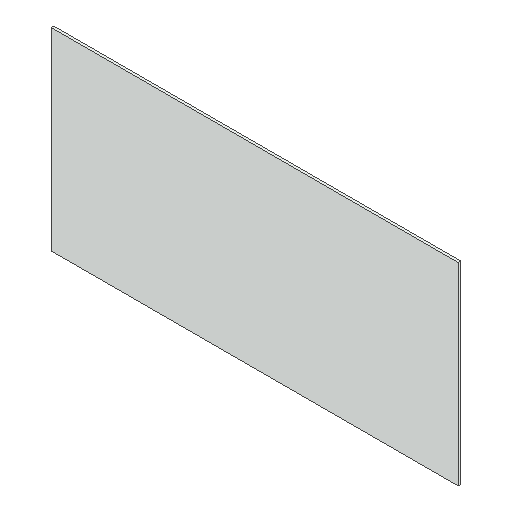
# Autodesk Inventor part: Chapa Frontal - Intake
Saved by Autodesk Inventor 2027.1 (Build 311270010, 270A)
## iProperties
Created: 2026-05-13
Part Number: Chapa Frontal - Intake
Material: Genérico
Document SubType Name: Modeling
Designer: djair.oliveira
Density: 1 g/cm^3
Appearance: Padrão
Author: djair.oliveira
Autodesk Inventor part; units mm, degrees
ref_plane "YZ Plane" through (0, 0, 0) normal (1, 0, 0) x (0, 1, 0)
ref_plane "XZ Plane" through (0, 0, 0) normal (0, 1, 0) x (-1, 0, 0)
ref_plane "XY Plane" through (0, 0, 0) normal (0, 0, 1) x (1, 0, 0)
sketch "Esboço1" plane through (0, 0, 0) normal (0, 0, 1) x (1, 0, 0)
  line L0 (315.675, -150) -> (-315.675, -150)
  line L1 (-315.675, -150) -> (-315.675, 150)
  line L2 (-315.675, 150) -> (315.675, 150)
  line L3 (315.675, 150) -> (315.675, -150)
  line L4 (315.675, -150) -> (-315.675, 150) construction
  line L5 (-315.675, -150) -> (315.675, 150) construction
  point P0 (0, 0)
  dimension "d0" = 631.35
  dimension "d1" = 300
  constraints: 12 end point, 2 midpoint, 2 parallel, 1 horizontal, 1 perpendicular
  measures "d0" distance of L0.start L0.end
  measures "d1" distance of L2.end L0.start
extrude "Extrusão1" add sketch "Esboço1" along normal blind 4
